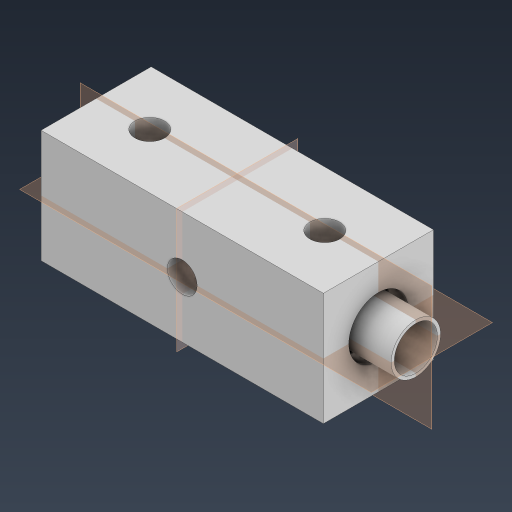
# Autodesk Inventor part: новое крепление штыря стрелялки
Saved by Autodesk Inventor 2023.2 (Build 272271030, 271C)
## iProperties
Created: 2025-09-05
Part Number: новое крепление штыря стрелялки
Material: Типовые
Document SubType Name: Modeling
Designer: Олег Коноваленко
Density: 1 g/cm^3
Appearance: По умолчанию
Author: Олег Коноваленко
Autodesk Inventor part; units mm, degrees
sketch "Эскиз1" plane through (0, 0, 0) normal (0, 1, 0) x (-1, 0, 0)
  line L0 (20, 7.8) -> (-20, 7.8)
  line L1 (-20, 7.8) -> (-20, -7.8)
  line L2 (-20, -7.8) -> (20, -7.8)
  line L3 (20, -7.8) -> (20, 7.8)
  line L4 (20, 7.8) -> (-20, -7.8) construction
  line L5 (-20, 7.8) -> (20, -7.8) construction
  point P0 (0, 0)
  dimension "d0" = 40
  dimension "d1" = 15.6
  constraints: 12 end point, 2 midpoint, 2 parallel, 1 horizontal, 1 perpendicular
  measures "d0" distance of L1.end L2.end
  measures "d1" distance of L2.end L0.start
extrude "Выдавливание1" add sketch "Эскиз1" along normal mid plane 16
sketch "Эскиз2" plane through (20, -8, -7.8) normal (1, 0, 0) x (0, 0, -1)
  circle A0 centre (-7.8, 8) radius 3.05
  dimension "d4" = 6.1
  constraints: 1 centre point, 1 coincident
  measures "d4" diameter of A0
extrude "Выдавливание2" cut sketch "Эскиз2" against normal up to next
sketch "Эскиз3" plane through (0, 8, 0) normal (0, 1, 0) x (1, 0, 0)
  circle A0 centre (-12.4, 0) radius 2.1
  circle A1 centre (12.4, 0) radius 2.1
  line L0 (28, 0) -> (-28, 0) projected
  line L1 (0, 10.92) -> (0, -10.92) projected
  line L2 (-20, 7.8) -> (-20, -7.8) projected
  line L3 (20, -7.8) -> (20, 7.8) projected
  point P0 (0, 0)
  dimension "d7" = 4.2
  dimension "d9" = 7.6
  dimension "d10" = 7.6
  constraints: 2 centre point, 2 point on line, 1 equal radius
  measures "d7" diameter of A0
  measures "d9" distance from line of L2 A0.centre
  measures "d10" distance from line of L3 A1.centre
extrude "Выдавливание3" cut sketch "Эскиз3" against normal blind 21.75
sketch "Эскиз4" plane through (-20, 8, 7.8) normal (0, 0, 1) x (1, 0, 0)
  circle A0 centre (20, -8) radius 2.1
  dimension "d13" = 4.2
  constraints: 1 centre point, 1 coincident
  measures "d13" diameter of A0
extrude "Выдавливание4" cut sketch "Эскиз4" against normal blind 19.55
sketch "Эскиз5" plane through (20, -8, -7.8) normal (1, 0, 0) x (0, 0, -1)
  circle A0 centre (-7.8, 8) radius 3.5
  circle A1 centre (-7.8, 8) radius 3.05 projected
  dimension "d17" = 7
  constraints: 1 centre point, 1 coincident
  measures "d17" diameter of A0
extrude "Выдавливание5" add sketch "Эскиз5" along normal blind 5.3
sketch "Эскиз6" plane through (20, -8, -7.8) normal (1, 0, 0) x (0, 0, -1)
  circle A0 centre (-7.8, 8) radius 3.5 projected
  circle A1 centre (-7.8, 8) radius 4.2
  dimension "d20" = 8.4
  constraints: 1 centre point, 1 coincident
  measures "d20" diameter of A1
extrude "Выдавливание6" cut sketch "Эскиз6" against normal blind 2.7
